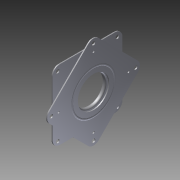
# Autodesk Inventor part: Triangle_3C
Saved by Autodesk Inventor 2014 (Build 180170000, 170)
## iProperties
Category: Miscellaneous
Company: Autodesk Inc.
Created: 2013-12-22
Part Number: Triangle_3C
Material: Generic
Document SubType Name: Modeling
Designer: Autodesk Inc.
Density: 1 g/cm^3
Description: Lazy Susan Bearing
Vendor: FIRSTChoice
Appearance: Default
Catalog Web Link: http://www.triangleoshkosh.com/assets/files/cad-drawings-lazy-susans/lazy-susan-3c.pdf
Author: Autodesk Inc.
Autodesk Inventor part; units mm, degrees
note: some values were not read from the file. Chosen so that the rebuilt part matches the saved one: direction of "Hole2".
ref_plane "XZ Plane" through (0, 0, 0) normal (0, 1, 0) x (-1, 0, 0)
sketch "Sketch1" plane through (0, 0, 0) normal (0, 0, 1) x (1, 0, 0)
  arc A0 (41.8853, -132.7525) -> (42.1663, -137.7917) centre (43.3819, -135.1965) ccw
  arc A1 (40.9995, -133.6037) -> (40.9995, -133.6037) centre (40.7786, -131.2035) ccw
  arc A2 (43.0328, -139.1543) -> (42.1663, -137.7917) centre (41.5281, -139.1543) ccw
  line L0 (43.0327, -141.4034) -> (43.0328, -139.1543)
  arc A3 (41.92, -139.5252) -> (41.4125, -138.6518) centre (40.9148, -139.5252) ccw
  arc A4 (40.6494, -128.2494) -> (41.1368, -128.7378) centre (41.2457, -128.1418) ccw
  arc A5 (41.8853, -132.7525) -> (41.1368, -128.7378) centre (40.7438, -130.8883) ccw
  arc A6 (41.3072, -131.8034) -> (40.937, -129.8311) centre (40.7438, -130.8883) ccw
  arc A7 (39.5318, -128.2494) -> (40.937, -129.8311) centre (41.2457, -128.1418) ccw
  line L1 (43.3819, -135.1965) -> (43.3819, -135.1965)
  line L2 (43.3819, -135.1965) -> (43.3819, -128.2495) construction
  arc A8 (44.5974, -137.7917) -> (44.8784, -132.7525) centre (43.3819, -135.1965) ccw
  arc A9 (45.7642, -133.6037) -> (45.7642, -133.6037) centre (45.9852, -131.2035) ccw
  arc A10 (44.5974, -137.7917) -> (43.7309, -139.1543) centre (45.2356, -139.1543) ccw
  line L3 (43.731, -141.4034) -> (43.7309, -139.1543)
  arc A11 (45.3512, -138.6518) -> (44.8437, -139.5252) centre (45.849, -139.5252) ccw
  line L4 (44.8437, -141.4034) -> (44.8437, -139.5252)
  line L5 (47.2319, -128.2494) -> (46.1143, -128.2494)
  arc A12 (45.627, -128.7378) -> (46.1143, -128.2494) centre (45.518, -128.1418) ccw
  arc A13 (45.627, -128.7378) -> (44.8784, -132.7525) centre (46.02, -130.8883) ccw
  arc A14 (45.8268, -129.8311) -> (45.4565, -131.8034) centre (46.02, -130.8883) ccw
  arc A15 (45.8268, -129.8311) -> (47.2319, -128.2494) centre (45.518, -128.1418) ccw
  arc A16 (45.3512, -138.6518) -> (45.4565, -131.8034) centre (43.3819, -135.1965) ccw
  arc A17 (43.3824, -141.8896) -> (43.731, -141.4034) centre (43.3373, -141.4892) ccw
  line L6 (43.3824, -141.8896) -> (42.4656, -141.8896)
  line L7 (41.8946, -139.6298) -> (40.9951, -139.6298)
  line L8 (40.9951, -139.6298) -> (40.9952, -141.6844)
  arc A18 (40.9952, -141.6844) -> (42.2182, -142.9074) centre (42.2182, -141.6843) ccw
  line L9 (42.2182, -142.9074) -> (43.3398, -142.9073)
  arc A19 (43.3398, -142.9073) -> (44.8437, -141.4034) centre (43.3398, -141.4034) ccw
  line L10 (39.3857, -158.5192) -> (47.3359, -158.5192) construction
  line L11 (41.92, -139.5252) -> (41.92, -141.4034)
  line L12 (41.8946, -139.6298) -> (41.8946, -141.3187)
  line L13 (41.92, -141.4034) -> (43.0327, -141.4034)
  arc A20 (41.8946, -141.3187) -> (42.4656, -141.8896) centre (42.4656, -141.3187) ccw
  line L14 (39.5318, -128.2494) -> (40.6494, -128.2494)
  arc A21 (41.3072, -131.8034) -> (41.4125, -138.6518) centre (43.3819, -135.1965) ccw
  point P0 (0, 0)
  point P1 (39.3972, -128.727)
  point P2 (47.3665, -128.727)
  dimension "d15" = 1.1127
  dimension "d39" = 1.1176
  dimension "d55" = 0.0254
  constraints: 48 point on circle, 30 end point, 22 centre point, 21 symmetric about line, 11 tangent, 4 parallel, 3 perpendicular, 2 vertical, 1 coincident, 1 horizontal, 9 other
  measures "d15" distance of L0.start L11.end
  measures "d39" distance of L14.start L14.end
  measures "d55" distance between parallel lines of L11 L12
revolve "Revolution1" add sketch "Sketch1" angle 360 about axis through (39.3857, -158.5192, 0) along (1, 0, 0) contours A0 A1 A21 A6 A7 A5 | A0 A2 L0 L13 L11 A3 A21 A1 | A1 A7 L14 A4 A5
revolve "Revolution2" add sketch "Sketch1" angle 360 about axis through (39.3857, -158.5192, 0) along (1, 0, 0) contours A8 A9 A16 A11 L4 A19 L9 A18 L8 L7 L12 A20 L6 A17 L3 A10 | A8 A13 A9 A15 A14 A16 | A13 A12 L5 A15 A9
ref_plane "Work Plane1" through (39.5318, -128.2494, 0) normal (1, 0, 0) x (0, 1, 0)
sketch "Sketch2" plane through (39.5318, -128.2494, 0) normal (1, 0, 0) x (0, 1, 0)
  circle A0 centre (-30.2699, 0) radius 30.2699 projected
  line L0 (7.8301, 38.1) -> (-68.3699, 38.1)
  line L1 (-68.3699, 38.1) -> (-68.3699, -38.1)
  line L2 (-68.3699, -38.1) -> (7.8301, -38.1)
  line L3 (7.8301, -38.1) -> (7.8301, 38.1)
  point P0 (128.2494, 0)
  point P1 (7.8301, 0)
  point P2 (-30.2699, -38.1)
  dimension "d82" = 76.2
  dimension "d83" = 76.2
  constraints: 8 end point, 2 midpoint, 2 parallel, 1 horizontal, 1 horizontal alignment, 1 perpendicular, 1 vertical alignment
  measures "d82" distance between parallel lines of L2 L0
  measures "d83" distance between parallel lines of L1 L3
extrude "Extrusion1" add sketch "Sketch2" along normal blind 1.1176
fillet "Fillet1" radius 7.9502 4 edges at (40.0906, -120.4192, 38.1) (40.0906, -120.4192, -38.1) (40.0906, -196.6192, 38.1) (40.0906, -196.6192, -38.1)
ref_plane "Work Plane2" through (47.2319, -128.2494, 0) normal (1, 0, 0) x (0, 1, 0)
sketch "Sketch3" plane through (47.2319, -128.2494, 0) normal (1, 0, 0) x (0, 1, 0)
  line L0 (-30.2699, 53.8815) -> (23.6117, 0)
  line L1 (23.6117, 0) -> (-30.2699, -53.8815)
  line L2 (-30.2699, -53.8815) -> (-84.1514, 0)
  line L3 (-84.1514, 0) -> (-30.2699, 53.8815)
  line L4 (7.8301, 30.1498) -> (7.8301, -30.1498) projected
  line L5 (-68.3699, -30.1498) -> (-68.3699, 30.1498) projected
  circle A0 centre (-30.2699, 0) radius 17.1158 projected
  point P0 (128.2494, 0)
  point P1 (7.8301, 0)
  point P2 (-68.3699, 0)
  dimension "d87" = 76.2
  constraints: 8 end point, 3 perpendicular, 2 horizontal alignment, 2 midpoint, 2 vertical alignment
  measures "d87" distance of L0.end L1.end
extrude "Extrusion2" add sketch "Sketch3" against normal up to surface (1.1176 mm away)
fillet "Fillet2" radius 7.9502 4 edges at (46.6731, -104.6377, 0) (46.6731, -158.5192, -53.8815) (46.6731, -158.5192, 53.8815) (46.6731, -212.4008, 0)
sketch "Sketch4" plane through (47.2319, -128.2494, 0) normal (1, 0, 0) x (0, 0, -1)
  line L0 (48.2599, -35.8915) -> (5.6216, -78.5297) projected
  line L1 (5.6216, 17.99) -> (48.2599, -24.6482) projected
  line L2 (-48.2599, -24.6482) -> (-5.6216, 17.99) projected
  line L3 (-5.6216, -78.5297) -> (-48.2599, -35.8915) projected
  point P0 (0, 128.2494)
  point P1 (-46.0328, -30.2699)
  point P2 (0, 15.7629)
  point P3 (46.0328, -30.2699)
  point P4 (0, -76.3026)
  point P5 (-38.1661, -30.2699)
  point P6 (0, 7.8962)
  point P7 (38.1661, -30.2699)
  point P8 (0, -68.4359)
  dimension "d91" = 65.1002
  dimension "d92" = 5.5499
  dimension "d93" = 65.1002
  dimension "d94" = 65.1002
  dimension "d95" = 65.1002
  dimension "d96" = 53.975
  dimension "d97" = 11.1125
  dimension "d98" = 5.5499
  dimension "d99" = 11.1125
  dimension "d100" = 53.975
  dimension "d101" = 11.1125
  dimension "d102" = 5.5499
  dimension "d103" = 5.5499
  dimension "d104" = 11.1125
  dimension "d105" = 11.1125
  dimension "d106" = 11.1125
  measures "d91" distance of point (46.033, -30.27) point (0, -76.303)
  measures "d92" distance from line of L1 point (46.033, -30.27)
  measures "d93" distance of point (0, 15.763) point (46.033, -30.27)
  measures "d94" distance of point (-46.033, -30.27) point (0, 15.763)
  measures "d95" distance of point (-46.033, -30.27) point (0, -76.303)
  measures "d96" distance of point (0, -68.436) point (38.166, -30.27)
  measures "d97" distance from line of L1 point (38.166, -30.27)
  measures "d98" distance from line of point (0, 15.763) L1
  measures "d99" distance from line of L1 point (0, 7.896)
  measures "d100" distance of point (-38.166, -30.27) point (0, 7.896)
  measures "d101" distance from line of L3 point (-38.166, -30.27)
  measures "d102" distance from line of L2 point (0, 15.763)
  measures "d103" distance from line of L3 point (-46.033, -30.27)
  measures "d104" distance from line of point (-38.166, -30.27) L2
  measures "d105" distance from line of point (0, -68.436) L0
  measures "d106" distance from line of L0 point (38.166, -30.27)
hole "Hole1" at (47.2319, -158.5192, 46.0328) at (47.2319, -112.4864, 0) at (47.2319, -158.5192, -46.0328) at (47.2319, -204.552, 0) direction (-1, 0, 0) diameter 3.9624 end through all
hole "Hole2" at (47.2319, -158.5192, 38.1661) at (47.2319, -120.3531, 0) at (47.2319, -158.5192, -38.1661) at (47.2319, -196.6853, 0) direction (-1, 0, 0) diameter 2.3876 end up to surface
sketch "Sketch5" plane through (40.6494, -128.2494, 0) normal (1, 0, 0) x (0, 0, -1)
  line L0 (30.1498, -68.3699) -> (-30.1498, -68.3699) projected
  line L1 (38.1, -0.1201) -> (38.1, -60.4197) projected
  line L2 (-30.1498, 7.8301) -> (30.1498, 7.8301) projected
  point P0 (0, 128.2494)
  point P1 (32.5501, 2.2802)
  point P2 (-32.5501, 2.2802)
  point P3 (-32.5501, -63.8412)
  point P4 (32.5501, -63.8412)
  dimension "d121" = 65.1002
  dimension "d122" = 5.5499
  dimension "d123" = 5.5499
  dimension "d124" = 4.5287
  constraints: 2 horizontal alignment, 2 vertical alignment
  measures "d121" distance of point (-32.55, 2.28) point (32.55, 2.28)
  measures "d122" distance from line of point (32.55, 2.28) L1
  measures "d123" distance from line of point (32.55, 2.28) L2
  measures "d124" distance from line of point (32.55, -63.841) L0
hole "Hole3" at (40.6494, -125.9691, -32.5501) at (40.6494, -125.9691, 32.5501) at (40.6494, -192.0905, 32.5501) at (40.6494, -192.0905, -32.5501) direction (-1, 0, 0) diameter 3.9624 end through all
equation "\"d15\" = d3"
equation "\"d93\" = d91"
equation "\"d94\" = d93"
equation "\"d95\" = d94"
equation "\"d98\" = d92"
equation "\"d99\" = d97"
equation "\"d100\" = d96"
equation "\"d101\" = d97"
equation "\"d102\" = d98"
equation "\"d103\" = d98"
equation "\"d104\" = d101"
equation "\"d105\" = d101"
equation "\"d106\" = d105"
equation "\"d123\" = d122"
equation "\"d8\" = d3"
equation "\"d3\" = 1.112684"
body "Solid1"
